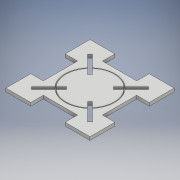
# Autodesk Inventor part: Zamek_I
Saved by Autodesk Inventor 2018 (Build 220112000, 112)
## iProperties
Created: 2018-10-19
Part Number: Zamek_I
Material: Ogólny
Document SubType Name: Modeling
Designer: EWA
Density: 1 g/cm^3
Appearance: Domyślna
Author: EWA
Autodesk Inventor part; units mm, degrees
ref_plane "YZ Plane" through (0, 0, 0) normal (1, 0, 0) x (0, 1, 0)
ref_plane "XZ Plane" through (0, 0, 0) normal (0, 1, 0) x (-1, 0, 0)
ref_plane "XY Plane" through (0, 0, 0) normal (0, 0, 1) x (1, 0, 0)
sketch "Szkic1" plane through (0, 0, 0) normal (0, 0, 1) x (1, 0, 0)
  line L0 (0, 0) -> (152, 0) construction
  line L1 (152, 0) -> (152, 152) construction
  line L2 (152, 152) -> (0, 152) construction
  line L3 (0, 152) -> (0, 0) construction
  line L4 (130, 22) -> (22, 22) construction
  line L5 (22, 22) -> (22, 130) construction
  line L6 (22, 130) -> (130, 130) construction
  line L7 (130, 130) -> (130, 22) construction
  line L8 (0, 0) -> (45, 0) construction
  line L9 (45, 0) -> (45, 45) construction
  line L10 (45, 45) -> (0, 45) construction
  line L11 (0, 45) -> (0, 0) construction
  line L12 (152, 0) -> (107, 0) construction
  line L13 (107, 0) -> (107, 45) construction
  line L14 (107, 45) -> (152, 45) construction
  line L15 (152, 45) -> (152, 0) construction
  line L16 (152, 152) -> (107, 152) construction
  line L17 (107, 152) -> (107, 107) construction
  line L18 (107, 107) -> (152, 107) construction
  line L19 (152, 107) -> (152, 152) construction
  line L20 (0, 152) -> (45, 152) construction
  line L21 (45, 152) -> (45, 107) construction
  line L22 (45, 107) -> (0, 107) construction
  line L23 (0, 107) -> (0, 152) construction
  line L24 (0, 0) -> (45, 0)
  line L25 (45, 0) -> (45, 22.5)
  line L26 (45, 22.5) -> (107, 22.5)
  line L27 (107, 22.5) -> (107, 0)
  line L28 (107, 0) -> (152, 0)
  line L29 (152, 0) -> (152, 45)
  line L30 (152, 45) -> (129.5, 45)
  line L31 (129.5, 45) -> (129.5, 107)
  line L32 (129.5, 107) -> (152, 107)
  line L33 (152, 107) -> (152, 152)
  line L34 (152, 152) -> (107, 152)
  line L35 (107, 152) -> (107, 129.5)
  line L36 (107, 129.5) -> (45, 129.5)
  line L37 (45, 129.5) -> (45, 152)
  line L38 (45, 152) -> (0, 152)
  line L39 (0, 152) -> (0, 107)
  line L40 (0, 107) -> (22.5, 107)
  line L41 (22.5, 107) -> (22.5, 45)
  line L42 (22.5, 45) -> (0, 45)
  line L43 (0, 45) -> (0, 0)
  line L44 (76, 129.5) -> (76, 76) construction
  circle A0 centre (76, 76) radius 45 construction
  line L45 (0, 152) -> (76, 76) construction
  line L46 (76, 76) -> (152, 0) construction
  line L47 (152, 152) -> (76, 76) construction
  line L48 (76, 76) -> (0, 0) construction
  line L49 (44.1802, 44.1802) -> (22.967, 22.967) construction
  line L50 (44.1802, 44.1802) -> (54.7868, 54.7868) construction
  line L51 (44.1802, 107.8198) -> (22.967, 129.033) construction
  line L52 (107.8198, 107.8198) -> (129.033, 129.033) construction
  line L53 (107.8198, 44.1802) -> (129.033, 22.967) construction
  line L54 (129.033, 129.033) -> (131.1543, 126.9117) construction
  line L55 (129.033, 129.033) -> (126.9117, 131.1543) construction
  line L56 (22.967, 129.033) -> (25.0883, 131.1543) construction
  line L57 (22.967, 129.033) -> (20.8457, 126.9117) construction
  line L58 (22.967, 22.967) -> (20.8457, 25.0883) construction
  line L59 (22.967, 22.967) -> (25.0883, 20.8457) construction
  line L60 (129.033, 22.967) -> (131.1543, 25.0883) construction
  line L61 (129.033, 22.967) -> (126.9117, 20.8457) construction
  line L62 (126.9117, 20.8457) -> (131.1543, 25.0883)
  line L63 (106.8058, 45.1942) -> (96.1992, 55.8008) construction
  arc A1 (109.8703, 46.3723) -> (109.8703, 105.6277) centre (76, 76) ccw
  line L64 (131.1543, 126.9117) -> (126.9117, 131.1543)
  line L65 (126.9117, 131.1543) -> (105.6277, 109.8703)
  line L66 (131.1543, 25.0883) -> (109.8703, 46.3723)
  arc A2 (105.6277, 109.8703) -> (46.3723, 109.8703) centre (76, 76) ccw
  arc A3 (42.1297, 105.6277) -> (42.1297, 46.3723) centre (76, 76) ccw
  arc A4 (46.3723, 42.1297) -> (105.6277, 42.1297) centre (76, 76) ccw
  circle A5 centre (76, 76) radius 43.5 construction
  line L67 (107.8198, 44.1802) -> (97.2132, 54.7868) construction
  line L68 (97.2132, 54.7868) -> (99.3345, 56.9081) construction
  line L69 (97.2132, 54.7868) -> (95.0919, 52.6655) construction
  line L70 (107.8198, 107.8198) -> (97.2132, 97.2132) construction
  line L71 (97.2132, 97.2132) -> (99.3345, 95.0919) construction
  line L72 (97.2132, 97.2132) -> (95.0919, 99.3345) construction
  line L73 (44.1802, 107.8198) -> (54.7868, 97.2132) construction
  line L74 (54.7868, 97.2132) -> (56.9081, 99.3345) construction
  line L75 (54.7868, 97.2132) -> (52.6655, 95.0919) construction
  line L76 (44.1802, 44.1802) -> (54.7868, 54.7868) construction
  line L77 (54.7868, 54.7868) -> (52.6655, 56.9081) construction
  line L78 (52.6655, 56.9081) -> (56.9081, 52.6655) construction
  line L79 (43.1928, 47.4354) -> (52.6655, 56.9081)
  line L80 (52.6655, 56.9081) -> (56.9081, 52.6655)
  line L81 (56.9081, 52.6655) -> (47.4354, 43.1928)
  line L82 (99.3345, 56.9081) -> (108.8072, 47.4354)
  line L83 (99.3345, 56.9081) -> (95.0919, 52.6655)
  line L84 (95.0919, 52.6655) -> (104.5646, 43.1928)
  line L85 (95.0919, 99.3345) -> (104.5646, 108.8072)
  line L86 (95.0919, 99.3345) -> (99.3345, 95.0919)
  line L87 (99.3345, 95.0919) -> (108.8072, 104.5646)
  line L88 (56.9081, 99.3345) -> (47.4354, 108.8072)
  line L89 (56.9081, 99.3345) -> (52.6655, 95.0919)
  line L90 (52.6655, 95.0919) -> (43.1928, 104.5646)
  arc A6 (108.8072, 47.4354) -> (108.8072, 104.5646) centre (76, 76) ccw
  arc A7 (47.4354, 43.1928) -> (104.5646, 43.1928) centre (76, 76) ccw
  arc A8 (43.1928, 104.5646) -> (43.1928, 47.4354) centre (76, 76) ccw
  arc A9 (104.5646, 108.8072) -> (47.4354, 108.8072) centre (76, 77.7417) ccw
  line L91 (105.6277, 42.1297) -> (126.9117, 20.8457)
  line L92 (109.8703, 105.6277) -> (131.1543, 126.9117)
  line L93 (46.3723, 42.1297) -> (25.0883, 20.8457)
  line L94 (25.0883, 20.8457) -> (20.8457, 25.0883)
  line L95 (20.8457, 25.0883) -> (42.1297, 46.3723)
  line L96 (42.1297, 105.6277) -> (20.8457, 126.9117)
  line L97 (20.8457, 126.9117) -> (25.0883, 131.1543)
  line L98 (25.0883, 131.1543) -> (46.3723, 109.8703)
  line L99 (76, 76) -> (119.5, 76) construction
  line L100 (76, 76) -> (129.5, 76) construction
  line L101 (121, 76) -> (129.5, 76) construction
  dimension "d11" = 90
  dimension "d35" = 1.5
  dimension "d0" = 152
  dimension "d1" = 152
  dimension "d2" = 22
  dimension "d3" = 45
  dimension "d4" = 45
  dimension "d5" = 45
  dimension "d6" = 45
  dimension "d7" = 45
  dimension "d8" = 45
  dimension "d9" = 45
  dimension "d10" = 45
  dimension "d12" = 30
  dimension "d14" = 30
  dimension "d16" = 30
  dimension "d18" = 30
  dimension "d20" = 3
  dimension "d21" = 3
  dimension "d22" = 3
  dimension "d23" = 3
  dimension "d24" = 3
  dimension "d25" = 3
  dimension "d36" = 15
  dimension "d37" = 3
  dimension "d38" = 3
  dimension "d39" = 15
  dimension "d40" = 3
  dimension "d41" = 3
  dimension "d42" = 15
  dimension "d43" = 3
  dimension "d44" = 3
  dimension "d45" = 15
  dimension "d46" = 3
  dimension "d47" = 6
  dimension "d50" = 43.5
  dimension "d51" = 8.5
  constraints: 204 end point, 25 perpendicular, 19 collinear, 18 point on circle, 17 point on line, 15 parallel, 10 midpoint, 8 centre point, 5 horizontal, 1 coincident, 1 vertical, 34 other
  measures "d0" distance of L2.end L1.end
  measures "d1" distance of L1.end L0.end
  measures "d2" distance between parallel lines of L0 L4
  measures "d3" distance of L10.end L9.end
  measures "d4" distance of L9.end L8.end
  measures "d5" distance of L13.end L14.end
  measures "d6" distance of L12.end L13.end
  measures "d7" distance of L18.end L17.end
  measures "d8" distance of L17.end L16.end
  measures "d9" distance of L21.end L22.end
  measures "d10" distance of L20.end L21.end
  measures "d12" distance of L49.start L49.end
  measures "d14" distance of L51.start L51.end
  measures "d16" distance of L52.start L52.end
  measures "d18" distance of L53.start L53.end
  measures "d20" distance of L52.end L54.end
  measures "d21" distance of L52.end L55.end
  measures "d22" distance of L51.end L56.end
  measures "d23" distance of L49.end L58.end
  measures "d24" distance of L49.end L59.end
  measures "d25" distance of L53.end L60.end
  measures "d36" distance of L53.start L67.end
  measures "d37" distance of L67.end L68.end
  measures "d38" distance of L67.end L69.end
  measures "d39" distance of L52.start L70.end
  measures "d40" distance of L70.end L71.end
  measures "d41" distance of L70.end L72.end
  measures "d42" distance of L51.start L73.end
  measures "d43" distance of L73.end L74.end
  measures "d44" distance of L73.end L75.end
  measures "d45" distance of L49.start L50.end
  measures "d46" distance of L50.end L77.end
  measures "d47" distance of L77.end L78.end
  measures "d50" distance of L99.start L99.end
  measures "d51" distance of L100.end L101.start
extrude "Wyciągnięcie proste1" add sketch "Szkic1" along normal blind 6
equation "\"d1\" = d0"
